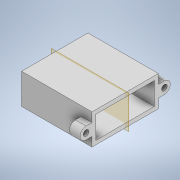
# Autodesk Inventor part: pudelko_baza
Saved by Autodesk Inventor 2021 (Build 250183000, 183)
## iProperties
Created: 2025-11-29
Part Number: pudelko_baza
Material: Generic
Document SubType Name: Modeling
Designer: huber
Density: 1 g/cm^3
Appearance: Default
Author: huber
Autodesk Inventor part; units mm, degrees
ref_plane "YZ Plane" through (0, 0, 0) normal (1, 0, 0) x (0, 1, 0)
ref_plane "XZ Plane" through (0, 0, 0) normal (0, 1, 0) x (-1, 0, 0)
sketch "Sketch2" plane through (0, 0, 0) normal (1, 0, 0) x (0, 1, 0)
  line L0 (23, 25) -> (0, 25)
  line L1 (0, 25) -> (0, -25)
  line L2 (0, -25) -> (23, -25)
  line L3 (23, -25) -> (23, 25)
  line L4 (20, 22) -> (3, 22)
  line L5 (3, 22) -> (3, -22)
  line L6 (3, -22) -> (20, -22)
  line L7 (20, -22) -> (20, 22)
  line L8 (0, -35) -> (0, 35) projected
  line L9 (-4.6, 0) -> (27.6, 0) projected
  point P0 (0, 0)
  dimension "d8" = 50
  dimension "d9" = 23
  dimension "d10" = 3
  dimension "d11" = 3
  dimension "d12" = 3
  dimension "d13" = 17
  constraints: 16 end point, 4 parallel, 2 horizontal, 2 perpendicular, 1 collinear, 2 other
  measures "d8" distance of L0.end L1.end
  measures "d9" distance of L1.end L2.end
  measures "d10" distance between parallel lines of L2 L6
  measures "d11" distance between parallel lines of L1 L5
  measures "d12" distance between parallel lines of L3 L7
  measures "d13" distance between parallel lines of L5 L7
extrude "Extrusion3" add sketch "Sketch2" along normal blind 3
extrude "Extrusion4" add sketch "Sketch2" along normal blind 53 contours L3 L9 L7 L4 L5 L1 L0 | L3 L2 L1 L9 L5 L6 L7
sketch "Sketch5" plane through (53, 0, 0) normal (1, 0, 0) x (0, 0, -1)
  line L0 (25, 0) -> (25, 23) projected
  line L1 (25, 23) -> (-25, 23) projected
  line L2 (-25, 23) -> (-25, 0) projected
  line L3 (-25, 0) -> (25, 0) projected
  line L4 (22, 3) -> (-22, 3) projected
  line L5 (-22, 3) -> (-22, 20) projected
  line L6 (-22, 20) -> (22, 20) projected
  line L7 (22, 20) -> (22, 3) projected
  line L8 (22, 11.5) -> (29.5, 11.5)
  line L9 (25, 0) -> (25, 23) projected
  circle A0 centre (29.5, 11.5) radius 4.5
  line L10 (29.5, 7) -> (25, 7)
  line L11 (29.5, 16) -> (25, 16)
  circle A1 centre (29.5, 11.5) radius 2.1
  point P0 (0, 0)
  dimension "d32" = 9
  dimension "d33" = 4.5
  dimension "d39" = 4.2
  constraints: 6 end point, 2 centre point, 2 coincident, 2 perpendicular, 2 point on circle, 2 point on line, 2 tangent, 1 horizontal, 1 midpoint
  measures "d32" diameter of A0
  measures "d33" distance from line of L0 L8.end
  measures "d39" diameter of A1
extrude "Extrusion7" add sketch "Sketch5" against normal blind 8 contours L0 A0 L10 | L0 L11 A0 | A0
sketch "Sketch6" plane through (45, 0, 0) normal (-1, 0, 0) x (0, 0, 1)
  line L0 (-29.5, 7) -> (-25, 7) projected
  line L1 (-25, 16) -> (-25, 7) projected
  line L2 (-25, 16) -> (-29.5, 16) projected
  arc A0 (-29.5, 16) -> (-29.5, 7) centre (-29.5, 11.5) ccw projected
  line L3 (-25.9204, 11.5) -> (-27.7102, 8.4)
  line L4 (-27.7102, 8.4) -> (-31.2898, 8.4)
  line L5 (-31.2898, 8.4) -> (-33.0796, 11.5)
  line L6 (-33.0796, 11.5) -> (-31.2898, 14.6)
  line L7 (-31.2898, 14.6) -> (-27.7102, 14.6)
  line L8 (-27.7102, 14.6) -> (-25.9204, 11.5)
  point P0 (0, 0)
  dimension "d36" = 6.2
  constraints: 12 end point, 1 coincident, 1 parallel, 13 other
  measures "d36" distance between parallel lines of L4 L7
extrude "Extrusion8" cut sketch "Sketch6" against normal blind 4 contours L3 L4 L5 L6 L7 L8
mirror "Mirror1" about plane through (0, 0, 0) normal (0, 0, 1) of "Extrusion7", "Extrusion8"
equation "\"d12\" = d11"
equation "\"d33\" = 0.5 * d32"
body "Solid2"
